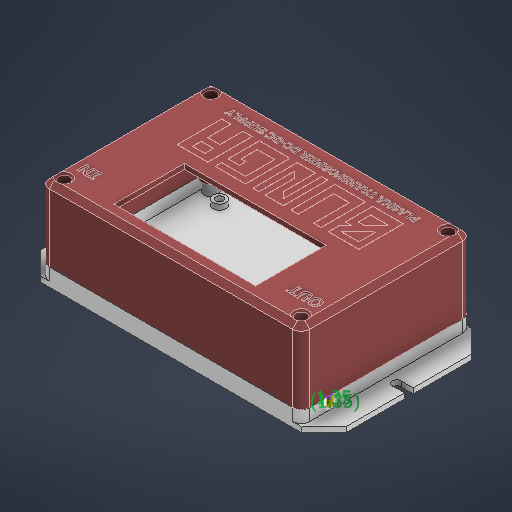
# Autodesk Inventor part: PowerSupplyCase-585W
Saved by Autodesk Inventor 2026.2 (Build 302298010, 298A)
## iProperties
Created: 2025-07-22
Part Number: PowerSupplyCase-585W
Material: Generic
Document SubType Name: Modeling
Designer: user
Density: 1 g/cm^3
Appearance: Default
Author: user
## iProperties of the stored document DrokSupplyCase_3DPrint.ipt
Created: 2025-07-22
Part Number: DrokSupplyCase_3DPrint
Material: Generic
Document SubType Name: Modeling
Designer: user
Density: 1 g/cm^3
Appearance: Default
Author: user
Autodesk Inventor part; units mm, degrees
(part 1 of 2)
sketch "Sketch1" plane through (0, 0, 0) normal (0, 1, 0) x (-1, 0, 0)
  line L0 (62, -35.75) -> (-62, -35.75) construction
  line L1 (-62, -35.75) -> (-62, 35.75) construction
  line L2 (-62, 35.75) -> (62, 35.75) construction
  line L3 (62, 35.75) -> (62, -35.75) construction
  line L4 (59, -32.775) -> (-59, -32.775) construction
  line L5 (-59, -32.775) -> (-59, 32.775) construction
  line L6 (-59, 32.775) -> (59, 32.775) construction
  line L7 (59, 32.775) -> (59, -32.775) construction
  circle A0 centre (59, -32.775) radius 2.1
  circle A1 centre (59, 32.775) radius 2.1
  circle A2 centre (-59, 32.775) radius 2.1
  circle A3 centre (-59, -32.775) radius 2.1
  circle A4 centre (59, -32.775) radius 3.75
  circle A5 centre (59, 32.775) radius 3.75
  circle A6 centre (-59, 32.775) radius 3.75
  circle A7 centre (-59, -32.775) radius 3.75
  line L8 (75, -43.75) -> (-75, -43.75)
  line L9 (-75, -43.75) -> (-75, 54.25)
  line L10 (-75, 54.25) -> (75, 54.25)
  line L11 (75, 54.25) -> (75, -43.75)
  line L12 (30.5, 5.75) -> (-48, 5.75)
  line L13 (-48, 5.75) -> (-48, 50.25)
  line L14 (-48, 50.25) -> (30.5, 50.25)
  line L15 (30.5, 50.25) -> (30.5, 5.75)
  line L16 (31.5, 21.85) -> (30.5, 21.85)
  line L17 (30.5, 21.85) -> (30.5, 34.15)
  line L18 (30.5, 34.15) -> (31.5, 34.15)
  line L19 (31.5, 34.15) -> (31.5, 21.85)
  line L20 (-48, 21.85) -> (-49, 21.85)
  line L21 (-49, 21.85) -> (-49, 34.15)
  line L22 (-49, 34.15) -> (-48, 34.15)
  line L23 (-48, 34.15) -> (-48, 21.85)
  line L24 (-72, -40.75) -> (72, -40.75)
  line L25 (72, -40.75) -> (72, 51.25)
  line L26 (72, 51.25) -> (-72, 51.25)
  line L27 (-72, 51.25) -> (-72, -40.75)
  line L28 (75, -43.75) -> (88, -30.75)
  line L29 (88, -30.75) -> (88, 41.25)
  line L30 (88, 41.25) -> (75, 54.25)
  circle A8 centre (81, 5.25) radius 2.5
  line L31 (81, 2.75) -> (88, 2.75)
  line L32 (81, 7.75) -> (88, 7.75)
  point P0 (0, 0)
  point P1 (0, -32.775)
  point P2 (0, -35.75)
  point P3 (-59, 0)
  point P4 (-62, 0)
  point P5 (30.5, 28)
  point P6 (-48, 28)
  point P7 (88, 5.25)
  point P8 (75, 5.25)
  dimension "d0" = 124
  dimension "d1" = 71.5
  dimension "d2" = 118
  dimension "d3" = 65.55
  dimension "d4" = 4.2
  dimension "d11" = 7.5
  dimension "d15" = 13
  dimension "d16" = 71.5
  dimension "d17" = 13
  dimension "d18" = 8
  dimension "d19" = 78.5
  dimension "d20" = 44.5
  dimension "d21" = 30
  dimension "d22" = 12.3
  dimension "d23" = 1
  dimension "d24" = 11
  dimension "d25" = 4
  dimension "d26" = 3
  dimension "d36" = 45
  dimension "d37" = 5
  dimension "d38" = 7
  dimension "d39" = 6
  constraints: 66 end point, 14 parallel, 10 midpoint, 9 centre point, 9 perpendicular, 8 coincident, 6 equal radius, 6 horizontal, 4 horizontal alignment, 2 equal length, 2 point on circle, 2 point on line, 2 tangent, 2 vertical alignment, 1 vertical, 3 other
  measures "d0" distance of L0.start L0.end
  measures "d1" distance of L2.end L0.start
  measures "d2" distance of L4.start L4.end
  measures "d3" distance of L6.end L4.start
  measures "d4" diameter of A0
  measures "d11" diameter of A4
  measures "d15" distance between parallel lines of L11 L3
  measures "d16" distance of L0.end L1.end
  measures "d17" distance between parallel lines of L9 L1
  measures "d18" distance between parallel lines of L8 L0
  measures "d19" distance of L12.start L12.end
  measures "d20" distance of L12.end L13.end
  measures "d21" distance between parallel lines of L12 L2
  measures "d22" distance of L18.end L16.start
  measures "d23" distance of L16.start L16.end
  measures "d24" distance between parallel lines of L5 L13
  measures "d25" distance between parallel lines of L10 L14
  measures "d26" distance between parallel lines of L8 L24
  measures "d36" angle of L28 L11
  measures "d37" diameter of A8
  measures "d38" distance of point (88, 5.25) A8.centre
  measures "d39" distance of point (75, 5.25) A8.centre
extrude "PCB Bosses" add sketch "Sketch1" along normal blind 6 contours A4 | A5 | A6 | A7
extrude "Floor" add sketch "Sketch1" along normal blind 3 contours A4 | A5 | A6 | A7 | L12 L13 L14 L15 | L15 L18 L19 L16 | L20 L21 L22 L13 | L27 L26 L25 L24
extrude "Fill in Holes" add sketch "Sketch1" along normal blind 1 contours A0 | A1 | A2 | A3
ref_plane "Work Plane1" through (-59, 49, -32.775) normal (0, 1, 0) x (1, 0, 0)
extrude "Wings" add sketch "Sketch1" along normal blind 3 contours L11 L30 L29 L32 A8 L31 L28
extrude "Bottom Wall" add sketch "Sketch1" along normal blind 3 contours L8 L9 L10 L11
mirror "Mirror1" about plane through (0, 0, 0) normal (1, 0, 0) of "Wings"
extrude "Bottom Wall 2" add sketch "Sketch1" along normal blind 10 contours L8 L9 L10 L11
fillet "Fillet1" radius 2 4 edges at (-72, 6.5, -40.75) (72, 6.5, -40.75) (-72, 6.5, 51.25) (72, 6.5, 51.25)
fillet "Fillet2" radius 5 4 edges at (-75, 6.5, 54.25) (75, 6.5, 54.25) (75, 6.5, -43.75) (-75, 6.5, -43.75)
sketch "Sketch2" plane through (0, 10, 0) normal (0, 1, 0) x (1, 0, 0)
  point P0 (0, 0)
sketch "Sketch3" plane through (0, 10, 0) normal (0, 1, 0) x (1, 0, 0)
  arc A0 (-70, 43.75) -> (-75, 38.75) centre (-70, 38.75) ccw projected
  line L0 (-75, 38.75) -> (-75, -49.25) projected
  arc A1 (-75, -49.25) -> (-70, -54.25) centre (-70, -49.25) ccw projected
  line L1 (-70, -54.25) -> (70, -54.25) projected
  arc A2 (70, -54.25) -> (75, -49.25) centre (70, -49.25) ccw projected
  line L2 (75, -49.25) -> (75, 38.75) projected
  arc A3 (75, 38.75) -> (70, 43.75) centre (70, 38.75) ccw projected
  line L3 (70, 43.75) -> (-70, 43.75) projected
  line L4 (72, 38.75) -> (72, -49.25) projected
  arc A4 (70, -51.25) -> (72, -49.25) centre (70, -49.25) ccw projected
  line L5 (70, -51.25) -> (-70, -51.25) projected
  arc A5 (-72, -49.25) -> (-70, -51.25) centre (-70, -49.25) ccw projected
  line L6 (-72, -49.25) -> (-72, 38.75) projected
  arc A6 (-70, 40.75) -> (-72, 38.75) centre (-70, 38.75) ccw projected
  line L7 (-70, 40.75) -> (70, 40.75) projected
  arc A7 (72, 38.75) -> (70, 40.75) centre (70, 38.75) ccw projected
  arc A8 (-70, 42.7) -> (-73.95, 38.75) centre (-70, 38.75) ccw
  line L8 (-70, 42.7) -> (70, 42.7)
  arc A9 (73.95, 38.75) -> (70, 42.7) centre (70, 38.75) ccw
  line L9 (73.95, 38.75) -> (73.95, -49.25)
  arc A10 (70, -53.2) -> (73.95, -49.25) centre (70, -49.25) ccw
  line L10 (70, -53.2) -> (-70, -53.2)
  arc A11 (-73.95, -49.25) -> (-70, -53.2) centre (-70, -49.25) ccw
  line L11 (-73.95, -49.25) -> (-73.95, 38.75)
  line L12 (70, 41.8) -> (-70, 41.8)
  arc A12 (-70, 41.8) -> (-73.05, 38.75) centre (-70, 38.75) ccw
  line L13 (-73.05, 38.75) -> (-73.05, -49.25)
  arc A13 (-73.05, -49.25) -> (-70, -52.3) centre (-70, -49.25) ccw
  line L14 (-70, -52.3) -> (70, -52.3)
  arc A14 (70, -52.3) -> (73.05, -49.25) centre (70, -49.25) ccw
  line L15 (73.05, -49.25) -> (73.05, 38.75)
  arc A15 (73.05, 38.75) -> (70, 41.8) centre (70, 38.75) ccw
  point P0 (0, 0)
  dimension "d48" = 1.05
  dimension "d49" = 1.05
  dimension "d50" = 0.9
  constraints: 16 end point, 16 point on circle, 8 centre point, 14 other
  measures "d48" radial gap between concentric circles of A0 A8
  measures "d49" distance between parallel lines of L7 L12
  measures "d50" distance between parallel lines of L12 L8
extrude "Lip 1" add sketch "Sketch3" along normal blind 1 contours L8 A9 L9 A10 L10 A11 L11 A8
sketch "Sketch4" plane through (-75, 3, -38.75) normal (-1, 0, 0) x (0, 0, 1)
  circle A0 centre (76.5, 3.35) radius 1.35
  line L0 (75.15, 2) -> (77.85, 2)
  line L1 (77.85, 2) -> (77.85, 8)
  line L2 (77.85, 8) -> (75.15, 8)
  line L3 (75.15, 8) -> (75.15, 2)
  line L4 (0, 8) -> (88, 8) projected
  line L5 (0, 7) -> (88, 7) projected
  line L6 (88, 7) -> (88, 0) projected
  line L7 (93, 0) -> (93, 7) projected
  point P0 (38.75, -3)
  point P1 (75.15, 3.35)
  point P2 (77.85, 3.35)
  dimension "d53" = 2.7
  dimension "d54" = 5
  dimension "d56" = 16.5
  constraints: 8 end point, 3 tangent, 2 parallel, 1 centre point, 1 collinear, 1 horizontal, 1 perpendicular
  measures "d53" diameter of A0
  measures "d54" distance between parallel lines of L5 L0
  measures "d56" distance from line of L7 A0.centre
sketch "Sketch5" plane through (0, 10, 0) normal (0, 1, 0) x (1, 0, 0)
  arc A0 (-70, 43.75) -> (-75, 38.75) centre (-70, 38.75) ccw projected
  line L0 (-75, 38.75) -> (-75, -49.25) projected
  arc A1 (-75, -49.25) -> (-70, -54.25) centre (-70, -49.25) ccw projected
  line L1 (-70, -54.25) -> (70, -54.25) projected
  arc A2 (70, -54.25) -> (75, -49.25) centre (70, -49.25) ccw projected
  line L2 (75, -49.25) -> (75, 38.75) projected
  arc A3 (75, 38.75) -> (70, 43.75) centre (70, 38.75) ccw projected
  line L3 (70, 43.75) -> (-70, 43.75) projected
  arc A4 (73.95, 38.75) -> (70, 42.7) centre (70, 38.75) ccw projected
  line L4 (73.95, 38.75) -> (73.95, -49.25) projected
  arc A5 (70, -53.2) -> (73.95, -49.25) centre (70, -49.25) ccw projected
  line L5 (70, -53.2) -> (-70, -53.2) projected
  arc A6 (-73.95, -49.25) -> (-70, -53.2) centre (-70, -49.25) ccw projected
  line L6 (-73.95, -49.25) -> (-73.95, 38.75) projected
  arc A7 (-70, 42.7) -> (-73.95, 38.75) centre (-70, 38.75) ccw projected
  line L7 (-70, 42.7) -> (70, 42.7) projected
  line L8 (70, 41.8) -> (-70, 41.8) projected
  arc A8 (-70, 41.8) -> (-73.05, 38.75) centre (-70, 38.75) ccw projected
  line L9 (-73.05, 38.75) -> (-73.05, -49.25) projected
  arc A9 (-73.05, -49.25) -> (-70, -52.3) centre (-70, -49.25) ccw projected
  line L10 (-70, -52.3) -> (70, -52.3) projected
  arc A10 (70, -52.3) -> (73.05, -49.25) centre (70, -49.25) ccw projected
  line L11 (73.05, -49.25) -> (73.05, 38.75) projected
  arc A11 (73.05, 38.75) -> (70, 41.8) centre (70, 38.75) ccw projected
  line L12 (72, 38.75) -> (72, -49.25) projected
  arc A12 (70, -51.25) -> (72, -49.25) centre (70, -49.25) ccw projected
  line L13 (70, -51.25) -> (-70, -51.25) projected
  arc A13 (-72, -49.25) -> (-70, -51.25) centre (-70, -49.25) ccw projected
  line L14 (-72, -49.25) -> (-72, 38.75) projected
  arc A14 (-70, 40.75) -> (-72, 38.75) centre (-70, 38.75) ccw projected
  line L15 (-70, 40.75) -> (70, 40.75) projected
  arc A15 (72, 38.75) -> (70, 40.75) centre (70, 38.75) ccw projected
  line L16 (-74.1, 38.75) -> (-74.1, -49.25)
  arc A16 (-74.1, -49.25) -> (-70, -53.35) centre (-70, -49.25) ccw
  line L17 (-70, -53.35) -> (70, -53.35)
  arc A17 (70, -53.35) -> (74.1, -49.25) centre (70, -49.25) ccw
  line L18 (74.1, -49.25) -> (74.1, 38.75)
  arc A18 (74.1, 38.75) -> (70, 42.85) centre (70, 38.75) ccw
  line L19 (70, 42.85) -> (-70, 42.85)
  arc A19 (-70, 42.85) -> (-74.1, 38.75) centre (-70, 38.75) ccw
  arc A20 (-70, 41.65) -> (-72.9, 38.75) centre (-70, 38.75) ccw
  line L20 (-70, 41.65) -> (70, 41.65)
  arc A21 (72.9, 38.75) -> (70, 41.65) centre (70, 38.75) ccw
  line L21 (72.9, 38.75) -> (72.9, -49.25)
  arc A22 (70, -52.15) -> (72.9, -49.25) centre (70, -49.25) ccw
  line L22 (70, -52.15) -> (-70, -52.15)
  arc A23 (-72.9, -49.25) -> (-70, -52.15) centre (-70, -49.25) ccw
  line L23 (-72.9, -49.25) -> (-72.9, 38.75)
  point P0 (0, 0)
  dimension "d59" = 0.15
  dimension "d60" = 0.15
  constraints: 16 end point, 16 point on circle, 8 centre point, 14 other
  measures "d59" radial gap between concentric circles of A7 A19
  measures "d60" radial gap between concentric circles of A8 A20
extrude "Extrusion10" add sketch "Sketch5" along normal blind 1.1 separate body contours L3 A3 L2 A2 L1 A1 L0 A0 | L20 A21 L21 A22 L22 A23 L23 A20
sketch "Sketch6" plane through (0, 11.1, 0) normal (0, 1, 0) x (1, 0, 0)
  line L0 (-75, 38.75) -> (-75, -49.25) projected
  arc A0 (-75, -49.25) -> (-70, -54.25) centre (-70, -49.25) ccw projected
  line L1 (-70, -54.25) -> (70, -54.25) projected
  arc A1 (70, -54.25) -> (75, -49.25) centre (70, -49.25) ccw projected
  line L2 (75, -49.25) -> (75, 38.75) projected
  arc A2 (75, 38.75) -> (70, 43.75) centre (70, 38.75) ccw projected
  line L3 (70, 43.75) -> (-70, 43.75) projected
  arc A3 (-70, 43.75) -> (-75, 38.75) centre (-70, 38.75) ccw projected
  arc A4 (-70, 42.85) -> (-74.1, 38.75) centre (-70, 38.75) ccw projected
  line L4 (-70, 42.85) -> (70, 42.85) projected
  arc A5 (74.1, 38.75) -> (70, 42.85) centre (70, 38.75) ccw projected
  line L5 (74.1, 38.75) -> (74.1, -49.25) projected
  arc A6 (70, -53.35) -> (74.1, -49.25) centre (70, -49.25) ccw projected
  line L6 (70, -53.35) -> (-70, -53.35) projected
  arc A7 (-74.1, -49.25) -> (-70, -53.35) centre (-70, -49.25) ccw projected
  line L7 (-74.1, -49.25) -> (-74.1, 38.75) projected
  line L8 (70, 41.65) -> (-70, 41.65) projected
  arc A8 (-70, 41.65) -> (-72.9, 38.75) centre (-70, 38.75) ccw projected
  line L9 (-72.9, 38.75) -> (-72.9, -49.25) projected
  arc A9 (-72.9, -49.25) -> (-70, -52.15) centre (-70, -49.25) ccw projected
  line L10 (-70, -52.15) -> (70, -52.15) projected
  arc A10 (70, -52.15) -> (72.9, -49.25) centre (70, -49.25) ccw projected
  line L11 (72.9, -49.25) -> (72.9, 38.75) projected
  arc A11 (72.9, 38.75) -> (70, 41.65) centre (70, 38.75) ccw projected
  line L12 (-70, 40.75) -> (70, 40.75) projected
  arc A12 (72, 38.75) -> (70, 40.75) centre (70, 38.75) ccw projected
  line L13 (72, 38.75) -> (72, -49.25) projected
  arc A13 (70, -51.25) -> (72, -49.25) centre (70, -49.25) ccw projected
  line L14 (70, -51.25) -> (-70, -51.25) projected
  arc A14 (-72, -49.25) -> (-70, -51.25) centre (-70, -49.25) ccw projected
  line L15 (-72, -49.25) -> (-72, 38.75) projected
  arc A15 (-70, 40.75) -> (-72, 38.75) centre (-70, 38.75) ccw projected
  point P0 (0, 0)
extrude "Extrusion11" add sketch "Sketch6" along normal up to surface (37.9 mm away) contours A3 L3 A2 L2 A1 L1 A0 L0 | L4 A5 L5 A6 L6 A7 L7 A4 | A11 L11 A10 L10 A9 L9 A8 L8 bodies 2
sketch "Sketch7" plane through (-70, 49, 54.25) normal (0, 1, 0) x (1, 0, 0)
  line L0 (39.5, 48.5) -> (118, 48.5) projected
  line L1 (39.5, 4) -> (39.5, 48.5) projected
  line L2 (118, 4) -> (39.5, 4) projected
  line L3 (118, 48.5) -> (118, 4) projected
  line L4 (119, 20.1) -> (118, 20.1) projected
  line L5 (119, 32.4) -> (119, 20.1) projected
  line L6 (118, 32.4) -> (119, 32.4) projected
  line L7 (39.5, 20.1) -> (38.5, 20.1) projected
  line L8 (38.5, 20.1) -> (38.5, 32.4) projected
  line L9 (38.5, 32.4) -> (39.5, 32.4) projected
  arc A0 (-2, 5) -> (0, 3) centre (0, 5) ccw projected
  line L10 (-2, 93) -> (-2, 5) projected
  arc A1 (0, 95) -> (-2, 93) centre (0, 93) ccw projected
  line L11 (140, 95) -> (0, 95) projected
  arc A2 (142, 93) -> (140, 95) centre (140, 93) ccw projected
  line L12 (142, 5) -> (142, 93) projected
  arc A3 (140, 3) -> (142, 5) centre (140, 5) ccw projected
  line L13 (0, 3) -> (140, 3) projected
  line L14 (-5, 5) -> (-5, 93) projected
  arc A4 (-5, 5) -> (0, 0) centre (0, 5) ccw projected
  line L15 (140, 0) -> (0, 0) projected
  arc A5 (140, 0) -> (145, 5) centre (140, 5) ccw projected
  line L16 (145, 93) -> (145, 5) projected
  arc A6 (145, 93) -> (140, 98) centre (140, 93) ccw projected
  line L17 (0, 98) -> (140, 98) projected
  arc A7 (0, 98) -> (-5, 93) centre (0, 93) ccw projected
  point P0 (70, 54.25)
extrude "Extrusion12" add sketch "Sketch7" along normal blind 3 contours L10 A1 L11 A2 L12 A3 L13 A0 | L14 A7 L17 A6 L16 A5 L15 A4 bodies 2
sketch "Sketch8" plane through (0, 3, 0) normal (0, 1, 0) x (1, 0, 0)
  circle A0 centre (-68.25, 37) radius 2.1
  circle A1 centre (-68.25, 37) radius 3.75
  circle A2 centre (59, -32.775) radius 3.75 projected
  circle A3 centre (59, 32.775) radius 3.75 projected
  circle A4 centre (-59, -32.775) radius 3.75 projected
  circle A5 centre (-59, 32.775) radius 3.75 projected
  arc A6 (70, -51.25) -> (72, -49.25) centre (70, -49.25) ccw projected
  line L0 (72, -49.25) -> (72, 38.75) projected
  arc A7 (72, 38.75) -> (70, 40.75) centre (70, 38.75) ccw projected
  line L1 (70, 40.75) -> (-70, 40.75) projected
  arc A8 (-70, 40.75) -> (-72, 38.75) centre (-70, 38.75) ccw projected
  line L2 (-72, 38.75) -> (-72, -49.25) projected
  arc A9 (-72, -49.25) -> (-70, -51.25) centre (-70, -49.25) ccw projected
  line L3 (-70, -51.25) -> (70, -51.25) projected
  line L4 (-70, 40.75) -> (70, 40.75) projected
  line L5 (-72, -49.25) -> (-72, 38.75) projected
  circle A10 centre (-68.25, -47.5) radius 2.1
  circle A11 centre (-68.25, -47.5) radius 3.75
  circle A12 centre (68.25, -47.5) radius 2.1
  circle A13 centre (68.25, -47.5) radius 3.75
  circle A14 centre (68.25, 37) radius 2.1
  circle A15 centre (68.25, 37) radius 3.75
  line L6 (70, -51.25) -> (-70, -51.25) projected
  line L7 (72, 38.75) -> (72, -49.25) projected
  point P0 (0, 0)
  dimension "d69" = 4.2
  dimension "d70" = 7.5
  constraints: 8 centre point, 8 tangent, 6 equal radius, 4 coincident
  measures "d69" diameter of A0
  measures "d70" diameter of A1
extrude "Extrusion13" add sketch "Sketch8" along normal up to surface (7 mm away) contours A1 | A15 | A11 | A13 bodies 1
sketch "Sketch9" plane through (-68.25, 3, -37) normal (0, 1, 0) x (1, 0, 0)
  circle A0 centre (0, 0) radius 2.1 projected
  circle A1 centre (136.5, 0) radius 2.1 projected
  circle A2 centre (136.5, -84.5) radius 2.1 projected
  circle A3 centre (0, -84.5) radius 2.1 projected
  point P0 (68.25, -37)
extrude "Extrusion14" cut sketch "Sketch9" against normal blind 2 bodies 1
extrude "Extrusion15" cut sketch "Sketch4" against normal up to surface (150 mm away) contours A0 | A0 L3 L5 L1 | L5 L3 L2 L1 bodies 1
sketch "Sketch10" plane through (-70, 52, 54.25) normal (0, 1, 0) x (1, 0, 0)
  arc A0 (1.75, 95) -> (-2, 91.25) centre (1.75, 91.25) ccw construction
  arc A1 (-2, 91.25) -> (1.75, 95) centre (1.75, 91.25) ccw construction
  circle A2 centre (1.75, 91.25) radius 2.1 construction
  circle A3 centre (138.25, 91.25) radius 2.1 construction
  arc A4 (138.25, 95) -> (142, 91.25) centre (138.25, 91.25) ccw construction
  arc A5 (142, 91.25) -> (138.25, 95) centre (138.25, 91.25) ccw construction
  circle A6 centre (138.25, 6.75) radius 2.1 construction
  arc A7 (142, 6.75) -> (138.25, 3) centre (138.25, 6.75) ccw construction
  arc A8 (138.25, 3) -> (142, 6.75) centre (138.25, 6.75) ccw construction
  arc A9 (1.75, 3) -> (-2, 6.75) centre (1.75, 6.75) ccw construction
  arc A10 (-2, 6.75) -> (1.75, 3) centre (1.75, 6.75) ccw construction
  circle A11 centre (1.75, 6.75) radius 2.1 construction
  circle A12 centre (1.75, 91.25) radius 1.7
  circle A13 centre (1.75, 91.25) radius 3.25
  circle A14 centre (1.75, 91.25) radius 5.25
  point P0 (70, 54.25)
  dimension "d81" = 3.4
  dimension "d82" = 6.5
  dimension "d83" = 2
  constraints: 3 centre point, 2 coincident
  measures "d81" diameter of A12
  measures "d82" diameter of A13
  measures "d83" radial gap between concentric circles of A13 A14
sketch "Sketch11" plane through (-70, 49, 54.25) normal (0, -1, 0) x (1, 0, 0)
  circle A0 centre (1.75, -91.25) radius 5.25 projected
  line L0 (-5, -93) -> (-5, -5) projected
  line L1 (-5, -93) -> (-5, -5) projected
  arc A1 (-5, -93) -> (0, -98) centre (0, -93) ccw projected
  line L2 (140, -98) -> (0, -98) projected
  line L3 (140, -98) -> (0, -98) projected
  line L4 (140, -95.9) -> (0, -95.9) projected
  arc A2 (140, -95.9) -> (142.9, -93) centre (140, -93) ccw projected
  line L5 (142.9, -5) -> (142.9, -93) projected
  arc A3 (142.9, -5) -> (140, -2.1) centre (140, -5) ccw projected
  line L6 (0, -2.1) -> (140, -2.1) projected
  arc A4 (0, -2.1) -> (-2.9, -5) centre (0, -5) ccw projected
  line L7 (-2.9, -93) -> (-2.9, -5) projected
  arc A5 (-2.9, -93) -> (0, -95.9) centre (0, -93) ccw projected
  line L8 (0, -95) -> (140, -95) projected
  arc A6 (-2, -93) -> (0, -95) centre (0, -93) ccw projected
  line L9 (-2, -5) -> (-2, -93) projected
  arc A7 (0, -3) -> (-2, -5) centre (0, -5) ccw projected
  line L10 (140, -3) -> (0, -3) projected
  arc A8 (142, -5) -> (140, -3) centre (140, -5) ccw projected
  line L11 (142, -93) -> (142, -5) projected
  arc A9 (140, -95) -> (142, -93) centre (140, -93) ccw projected
  arc A10 (-5, -93) -> (0, -98) centre (0, -93) ccw projected
  point P0 (70, -54.25)
  point P1 (5.4242, -95)
  point P2 (-2, -87.5758)
extrude "TopMount1" add sketch "Sketch11" along normal up to surface (39 mm away) contours A0 L8 A6 L9 bodies 2
extrude "TopMount2" cut sketch "Sketch10" against normal up to surface (42 mm away) contours A12 bodies 2
ref_plane "Work Plane2" through (0, 12, 0) normal (0, -1, 0) x (1, 0, 0)
extrude "TopMount3" cut sketch "Sketch10" against normal up to surface (40 mm away) contours A13 bodies 2
ref_plane "Work Plane3" through (0, 10, 49.25) normal (1, 0, 0) x (0, 0, -1)
ref_plane "Work Plane4" through (-70, 10, 5.25) normal (0, 0, 1) x (1, 0, 0)
mirror "Mirror2" about plane through (0, 10, 49.25) normal (1, 0, 0) of "TopMount3", "TopMount2", "TopMount1" bodies 2
mirror "Mirror3" about plane through (-70, 10, 5.25) normal (0, 0, 1) of "TopMount3", "TopMount2", "TopMount1", "Mirror2" bodies 2
sketch "Sketch12" plane through (-70, 52, 54.25) normal (0, 1, 0) x (1, 0, 0)
  line L0 (78.75, 56) -> (61.25, 56) construction
  line L1 (61.25, 56) -> (61.25, 81.5) construction
  line L2 (61.25, 81.5) -> (78.75, 81.5) construction
  line L3 (78.75, 81.5) -> (78.75, 56) construction
  line L4 (57, 56) -> (39.5, 56) construction
  line L5 (57, 81.5) -> (57, 56) construction
  line L6 (39.5, 81.5) -> (57, 81.5) construction
  line L7 (39.5, 56) -> (39.5, 81.5) construction
  line L8 (35.25, 56) -> (17.75, 56) construction
  line L9 (35.25, 81.5) -> (35.25, 56) construction
  line L10 (17.75, 81.5) -> (35.25, 81.5) construction
  line L11 (17.75, 56) -> (17.75, 81.5) construction
  line L12 (100.5, 56) -> (83, 56) construction
  line L13 (100.5, 81.5) -> (100.5, 56) construction
  line L14 (83, 81.5) -> (100.5, 81.5) construction
  line L15 (83, 56) -> (83, 81.5) construction
  line L16 (78.75, 56) -> (61.25, 56) construction
  line L17 (78.75, 81.5) -> (78.75, 56) construction
  line L18 (61.25, 81.5) -> (78.75, 81.5) construction
  line L19 (61.25, 56) -> (61.25, 81.5) construction
  line L20 (57, 56) -> (39.5, 56) construction
  line L21 (57, 81.5) -> (57, 56) construction
  line L22 (39.5, 81.5) -> (57, 81.5) construction
  line L23 (39.5, 56) -> (39.5, 81.5) construction
  line L24 (122.25, 56) -> (104.75, 56) construction
  line L25 (122.25, 81.5) -> (122.25, 56) construction
  line L26 (104.75, 81.5) -> (122.25, 81.5) construction
  line L27 (104.75, 56) -> (104.75, 81.5) construction
  line L28 (100.5, 56) -> (83, 56) construction
  line L29 (100.5, 81.5) -> (100.5, 56) construction
  line L30 (83, 81.5) -> (100.5, 81.5) construction
  line L31 (83, 56) -> (83, 81.5) construction
  line L32 (78.75, 56) -> (61.25, 56) construction
  line L33 (78.75, 81.5) -> (78.75, 56) construction
  line L34 (61.25, 81.5) -> (78.75, 81.5) construction
  line L35 (61.25, 56) -> (61.25, 81.5) construction
  line L36 (78.75, 81.5) -> (78.75, 56)
  line L37 (68.25, 56) -> (68.25, 73)
  line L38 (68.25, 73) -> (64.75, 76.5)
  line L39 (64.75, 76.5) -> (64.75, 56)
  line L40 (61.25, 56) -> (61.25, 81.5)
  line L41 (61.25, 81.5) -> (71.75, 81.5)
  line L42 (71.75, 81.5) -> (71.75, 63.25)
  line L43 (71.75, 63.25) -> (75.25, 59.75)
  line L44 (75.25, 59.75) -> (75.25, 81.5)
  line L45 (75.25, 81.5) -> (78.75, 81.5)
  line L46 (39.5, 56) -> (57, 56)
  line L47 (57, 56) -> (57, 81.5)
  line L48 (57, 81.5) -> (39.5, 81.5)
  line L49 (39.5, 81.5) -> (39.5, 63.5)
  line L50 (39.5, 63.5) -> (46, 63.5)
  line L51 (46, 63.5) -> (46, 67.25)
  line L52 (46, 67.25) -> (43.25, 67.25)
  line L53 (43.25, 67.25) -> (43.25, 76.5)
  line L54 (43.25, 76.5) -> (53.25, 76.5)
  line L55 (53.25, 76.5) -> (53.25, 59.75)
  line L56 (53.25, 59.75) -> (39.5, 59.75)
  line L57 (39.5, 59.75) -> (39.5, 56)
  line L58 (35.25, 81.5) -> (30, 81.5)
  line L59 (30, 81.5) -> (30, 68.25)
  line L60 (30, 68.25) -> (23, 68.25)
  line L61 (23, 68.25) -> (23, 81.5)
  line L62 (23, 81.5) -> (17.75, 81.5)
  line L63 (17.75, 81.5) -> (17.75, 56)
  line L64 (17.75, 56) -> (35.25, 56)
  line L65 (35.25, 56) -> (35.25, 81.5)
  line L66 (30, 59.5) -> (30, 64.5)
  line L67 (30, 64.5) -> (23, 64.5)
  line L68 (23, 64.5) -> (23, 59.5)
  line L69 (23, 59.5) -> (30, 59.5)
  line L70 (100.5, 56) -> (96.25, 56)
  line L71 (96.25, 56) -> (96.25, 76.5)
  line L72 (96.25, 76.5) -> (87.25, 76.5)
  line L73 (87.25, 76.5) -> (87.25, 56)
  line L74 (83, 56) -> (83, 81.5)
  line L75 (83, 81.5) -> (100.5, 81.5)
  line L76 (100.5, 81.5) -> (100.5, 56)
  line L77 (122.25, 56) -> (122.25, 81.5)
  line L78 (122.25, 81.5) -> (104.75, 81.5)
  line L79 (104.75, 56) -> (122.25, 56)
  line L80 (118.5, 59.75) -> (118.5, 69.031)
  line L81 (118.5, 64.3905) -> (111.5898, 64.3905) construction
  line L82 (107.3101, 68.75) -> (104.75, 68.75) construction
  line L83 (118.5, 69.031) -> (117.1257, 69.031)
  line L84 (117.1257, 69.031) -> (108.5, 60.4053)
  line L85 (117.1257, 69.031) -> (129.3242, 69.031) construction
  line L86 (108.5, 60.4053) -> (108.5, 59.75)
  line L87 (108.5, 59.75) -> (118.5, 59.75)
  line L88 (107.3101, 68.75) -> (104.75, 68.75) construction
  line L89 (112.25, 69.4886) -> (108.5, 69.4886)
  line L90 (108.5, 69.4886) -> (108.5, 76.5)
  line L91 (108.5, 76.5) -> (118.5, 76.5)
  line L92 (118.5, 76.5) -> (118.5, 75.7386)
  line L93 (118.5, 75.7386) -> (112.25, 69.4886)
  line L94 (118.5, 75.7386) -> (125.6277, 75.7386) construction
  line L95 (104.75, 56) -> (104.75, 61.9886)
  line L96 (104.75, 61.9886) -> (108.5, 65.7386)
  line L97 (108.5, 65.7386) -> (104.75, 65.7386)
  line L98 (104.75, 81.5) -> (104.75, 65.7386)
  line L99 (108.5, 65.7386) -> (112.25, 69.4886) construction
  line L100 (5, 93) -> (135, 93) projected
  line L101 (70, 93) -> (70, 48.5) construction
  line L102 (39.5, 48.5) -> (118, 48.5) construction
  line L103 (61.25, 56) -> (64.75, 56)
  line L104 (68.25, 56) -> (78.75, 56)
  line L105 (83, 56) -> (87.25, 56)
  point P0 (70, 54.25)
  point P1 (70, 68.75)
  point P2 (60, 68.75)
  point P3 (70, 56)
  point P4 (61.25, 68.75)
  point P5 (48.25, 56)
  point P6 (48.25, 68.75)
  point P7 (39.5, 68.75)
  point P8 (26.5, 56)
  point P9 (26.5, 68.75)
  point P10 (17.75, 68.75)
  point P11 (91.75, 56)
  point P12 (91.75, 68.75)
  point P13 (83, 68.75)
  point P14 (70, 56)
  point P15 (70, 68.75)
  point P16 (61.25, 68.75)
  point P17 (48.25, 56)
  point P18 (48.25, 68.75)
  point P19 (39.5, 68.75)
  point P20 (113.5, 56)
  point P21 (113.5, 68.75)
  point P22 (91.75, 56)
  point P23 (91.75, 68.75)
  point P24 (83, 68.75)
  point P25 (70, 56)
  point P26 (70, 68.75)
  point P27 (61.25, 68.75)
  point P28 (107.3101, 68.75)
  point P29 (102.125, 63.5649)
  point P30 (70, 68.75)
  point P31 (70, 70.75)
  point P32 (5, 91.25)
  point P33 (135, 91.25)
  point P34 (70, 70.75)
  constraints: 208 end point, 27 perpendicular, 18 point on line, 17 collinear, 9 horizontal, 6 midpoint, 6 vertical, 4 parallel, 3 horizontal alignment, 2 coincident, 2 vertical alignment, 1 equal length, 6 other
extrude "Extrusion19" cut sketch "Sketch12" against normal blind 0.1 bodies 2
sketch "Sketch13" plane through (-70, 52, 54.25) normal (0, 1, 0) x (1, 0, 0)
  line L0 (139.3009, 14) -> (124.6991, 14) construction
  line L1 (124.6991, 14) -> (124.6991, 17.3208) construction
  line L2 (124.6991, 17.3208) -> (139.3009, 17.3208) construction
  line L3 (139.3009, 17.3208) -> (139.3009, 14) construction
  line L4 (141.5993, 14) -> (126.9975, 14) construction
  line L5 (126.9975, 14) -> (126.9975, 17.3208) construction
  line L6 (126.9975, 17.3208) -> (141.5993, 17.3208) construction
  line L7 (141.5993, 17.3208) -> (141.5993, 14) construction
  line L8 (11.2814, 14) -> (-3.3204, 14) construction
  line L9 (-3.3204, 14) -> (-3.3204, 17.3208) construction
  line L10 (-3.3204, 17.3208) -> (11.2814, 17.3208) construction
  line L11 (11.2814, 17.3208) -> (11.2814, 14) construction
  line L12 (140, 91.25) -> (140, 6.75) projected
  line L13 (134, 5) -> (117.75, 5) projected
  line L14 (136.0195, 85.116) -> (3.9805, 85.116) construction
  line L15 (3.9805, 85.116) -> (3.9805, 87.6939) construction
  line L16 (3.9805, 87.6939) -> (136.0195, 87.6939) construction
  line L17 (136.0195, 87.6939) -> (136.0195, 85.116) construction
  line L18 (6, 93) -> (134, 93) projected
  spline S0 degree 2 poles (133.2239, 17.1235) (133.2239, 18.5808) (134.7784, 20.247) (136.1288, 20.247) knots 0 0 0 1 2 2 2
  spline S1 degree 2 poles (136.1288, 20.247) (137.4841, 20.247) (139.0289, 18.5614) (139.0289, 17.1235) knots 0 0 0 1 2 2 2
  spline S2 degree 2 poles (139.0289, 17.1235) (139.0289, 15.6808) (137.4841, 14) (136.1288, 14) knots 0 0 0 1 2 2 2
  spline S3 degree 2 poles (136.1288, 14) (134.7784, 14) (133.2239, 15.671) (133.2239, 17.1235) knots 0 0 0 1 2 2 2
  spline S4 degree 2 poles (134.7784, 17.1235) (134.7784, 16.5843) (134.997, 15.8314) (135.1865, 15.5933) knots 0 0 0 1 2 2 2
  spline S5 degree 2 poles (135.1865, 15.5933) (135.3759, 15.3456) (135.8617, 15.1318) (136.124, 15.1318) knots 0 0 0 1 2 2 2
  spline S6 degree 2 poles (136.124, 15.1318) (136.4009, 15.1318) (136.8526, 15.331) (137.0615, 15.5836) knots 0 0 0 1 2 2 2
  spline S7 degree 2 poles (137.0615, 15.5836) (137.2461, 15.8168) (137.4744, 16.5892) (137.4744, 17.1235) knots 0 0 0 1 2 2 2
  spline S8 degree 2 poles (137.4744, 17.1235) (137.4744, 17.6773) (137.2558, 18.4059) (137.0664, 18.6537) knots 0 0 0 1 2 2 2
  spline S9 degree 2 poles (137.0664, 18.6537) (136.8769, 18.9014) (136.3863, 19.1152) (136.124, 19.1152) knots 0 0 0 1 2 2 2
  spline S10 degree 2 poles (136.124, 19.1152) (135.8568, 19.1152) (135.3613, 18.8868) (135.1816, 18.644) knots 0 0 0 1 2 2 2
  spline S11 degree 2 poles (135.1816, 18.644) (134.9873, 18.3816) (134.7784, 17.687) (134.7784, 17.1235) knots 0 0 0 1 2 2 2
  spline S12 degree 2 poles (129.9061, 20.247) (131.1157, 20.247) (132.4176, 19.0812) (132.4176, 17.9542) knots 0 0 0 1 2 2 2
  line L19 (132.4176, 17.9542) -> (132.4176, 14.1263)
  line L20 (132.4176, 14.1263) -> (130.9117, 14.1263)
  line L21 (130.9117, 14.1263) -> (130.9117, 17.8667)
  spline S13 degree 2 poles (130.9117, 17.8667) (130.9117, 18.4934) (130.4405, 19.1054) (129.9061, 19.1054) knots 0 0 0 1 2 2 2
  spline S14 degree 2 poles (129.9061, 19.1054) (129.3864, 19.1054) (128.9006, 18.5177) (128.9006, 17.8667) knots 0 0 0 1 2 2 2
  line L22 (128.9006, 17.8667) -> (128.9006, 14.1263)
  line L23 (128.9006, 14.1263) -> (127.3947, 14.1263)
  line L24 (127.3947, 14.1263) -> (127.3947, 17.9493)
  spline S15 degree 2 poles (127.3947, 17.9493) (127.3947, 19.0569) (128.6626, 20.247) (129.9061, 20.247) knots 0 0 0 1 2 2 2
  line L25 (125.0873, 20.1207) -> (125.0873, 15.2679)
  line L26 (125.0873, 15.2679) -> (126.8604, 15.2679)
  line L27 (126.8604, 15.2679) -> (126.8604, 14.1263)
  line L28 (126.8604, 14.1263) -> (121.8084, 14.1263)
  line L29 (121.8084, 14.1263) -> (121.8084, 15.2679)
  line L30 (121.8084, 15.2679) -> (123.5814, 15.2679)
  line L31 (123.5814, 15.2679) -> (123.5814, 20.1207)
  line L32 (123.5814, 20.1207) -> (125.0873, 20.1207)
  line L33 (7.677, 19.9944) -> (10.9025, 19.9944)
  line L34 (10.9025, 19.9944) -> (10.9025, 18.95)
  line L35 (10.9025, 18.95) -> (10.0427, 18.95)
  line L36 (10.0427, 18.95) -> (10.0427, 15.0444)
  line L37 (10.0427, 15.0444) -> (10.9025, 15.0444)
  line L38 (10.9025, 15.0444) -> (10.9025, 14)
  line L39 (10.9025, 14) -> (7.677, 14)
  line L40 (7.677, 14) -> (7.677, 15.0444)
  line L41 (7.677, 15.0444) -> (8.5368, 15.0444)
  line L42 (8.5368, 15.0444) -> (8.5368, 18.95)
  line L43 (8.5368, 18.95) -> (7.677, 18.95)
  line L44 (7.677, 18.95) -> (7.677, 19.9944)
  line L45 (1.5417, 19.9944) -> (2.9893, 19.9944)
  line L46 (2.9893, 19.9944) -> (5.3016, 15.8168)
  line L47 (5.3016, 15.8168) -> (5.3016, 19.9944)
  line L48 (5.3016, 19.9944) -> (6.6763, 19.9944)
  line L49 (6.6763, 19.9944) -> (6.6763, 14)
  line L50 (6.6763, 14) -> (4.8304, 14)
  line L51 (4.8304, 14) -> (2.9165, 17.4344)
  line L52 (2.9165, 17.4344) -> (2.9165, 14)
  line L53 (2.9165, 14) -> (1.5417, 14)
  line L54 (1.5417, 14) -> (1.5417, 19.9944)
  spline S16 degree 2 poles (121.2823, 86.4571) (121.2823, 86.735) (121.4601, 87.2392) (121.6249, 87.4072) knots 0 0 0 1 2 2 2
  spline S17 degree 2 poles (121.6249, 87.4072) (121.7251, 87.5139) (121.9707, 87.6884) (122.1161, 87.7498) knots 0 0 0 1 2 2 2
  spline S18 degree 2 poles (122.1161, 87.7498) (122.2647, 87.8112) (122.6105, 87.8823) (122.8238, 87.8823) knots 0 0 0 1 2 2 2
  line L55 (122.8238, 87.8823) -> (123.3473, 87.8823)
  line L56 (123.3473, 87.8823) -> (123.3473, 89.1878)
  line L57 (123.3473, 89.1878) -> (124.3491, 89.1878)
  line L58 (124.3491, 89.1878) -> (124.3491, 85.2)
  line L59 (124.3491, 85.2) -> (122.8012, 85.2)
  spline S19 degree 2 poles (122.8012, 85.2) (122.4586, 85.2) (121.9577, 85.3261) (121.7541, 85.4618) knots 0 0 0 1 2 2 2
  spline S20 degree 2 poles (121.7541, 85.4618) (121.5279, 85.6137) (121.2823, 86.1113) (121.2823, 86.4571) knots 0 0 0 1 2 2 2
  spline S21 degree 2 poles (122.31, 86.483) (122.31, 86.3117) (122.4716, 86.0693) (122.5814, 86.0241) knots 0 0 0 1 2 2 2
  spline S22 degree 2 poles (122.5814, 86.0241) (122.7236, 85.9627) (122.9822, 85.9433) (123.2051, 85.9433) knots 0 0 0 1 2 2 2
  line L60 (123.2051, 85.9433) -> (123.3473, 85.9433)
  line L61 (123.3473, 85.9433) -> (123.3473, 87.139)
  line L62 (123.3473, 87.139) -> (123.2762, 87.139)
  spline S23 degree 2 poles (123.2762, 87.139) (123.1373, 87.139) (122.8852, 87.1325) (122.7915, 87.1164) knots 0 0 0 1 2 2 2
  spline S24 degree 2 poles (122.7915, 87.1164) (122.7107, 87.1034) (122.533, 87.0259) (122.4845, 86.9774) knots 0 0 0 1 2 2 2
  spline S25 degree 2 poles (122.4845, 86.9774) (122.3811, 86.8805) (122.31, 86.6639) (122.31, 86.483) knots 0 0 0 1 2 2 2
  line L63 (118.0863, 89.1878) -> (120.7459, 89.1878)
  line L64 (120.7459, 89.1878) -> (120.7459, 85.2)
  line L65 (120.7459, 85.2) -> (119.7441, 85.2)
  line L66 (119.7441, 85.2) -> (119.7441, 88.4284)
  line L67 (119.7441, 88.4284) -> (118.0863, 88.4284)
  line L68 (118.0863, 88.4284) -> (118.0863, 89.1878)
  line L69 (118.0378, 89.1878) -> (116.6902, 85.2)
  line L70 (116.6902, 85.2) -> (115.5979, 85.2)
  line L71 (115.5979, 85.2) -> (114.2504, 89.1878)
  line L72 (114.2504, 89.1878) -> (115.2812, 89.1878)
  line L73 (115.2812, 89.1878) -> (115.5301, 88.3735)
  line L74 (115.5301, 88.3735) -> (116.7839, 88.3735)
  line L75 (116.7839, 88.3735) -> (117.036, 89.1878)
  line L76 (117.036, 89.1878) -> (118.0378, 89.1878)
  line L77 (115.7498, 87.6496) -> (116.157, 86.3311)
  line L78 (116.157, 86.3311) -> (116.5674, 87.6496)
  line L79 (116.5674, 87.6496) -> (115.7498, 87.6496)
  spline S26 degree 2 poles (112.6216, 89.2589) (113.0805, 89.2589) (113.7721, 89.0812) (114.0694, 88.9519) knots 0 0 0 1 2 2 2
  line L80 (114.0694, 88.9519) -> (114.0694, 88.0018)
  line L81 (114.0694, 88.0018) -> (113.9789, 88.0018)
  spline S27 degree 2 poles (113.9789, 88.0018) (113.6784, 88.2571) (112.9577, 88.5318) (112.6184, 88.5318) knots 0 0 0 1 2 2 2
  spline S28 degree 2 poles (112.6184, 88.5318) (112.5311, 88.5318) (112.25, 88.493) (112.166, 88.4542) knots 0 0 0 1 2 2 2
  spline S29 degree 2 poles (112.166, 88.4542) (112.0626, 88.409) (111.9171, 88.2442) (111.9171, 88.1117) knots 0 0 0 1 2 2 2
  spline S30 degree 2 poles (111.9171, 88.1117) (111.9171, 87.9598) (112.153, 87.7724) (112.3146, 87.7304) knots 0 0 0 1 2 2 2
  spline S31 degree 2 poles (112.3146, 87.7304) (112.5182, 87.6754) (112.9803, 87.5817) (113.1839, 87.5106) knots 0 0 0 1 2 2 2
  spline S32 degree 2 poles (113.1839, 87.5106) (113.646, 87.349) (114.0468, 86.7964) (114.0468, 86.3828) knots 0 0 0 1 2 2 2
  spline S33 degree 2 poles (114.0468, 86.3828) (114.0468, 85.8237) (113.0999, 85.1289) (112.389, 85.1289) knots 0 0 0 1 2 2 2
  spline S34 degree 2 poles (112.389, 85.1289) (112.0335, 85.1289) (111.329, 85.2743) (111.0511, 85.3971) knots 0 0 0 1 2 2 2
  line L82 (111.0511, 85.3971) -> (111.0511, 86.3085)
  line L83 (111.0511, 86.3085) -> (111.1383, 86.3085)
  spline S35 degree 2 poles (111.1383, 86.3085) (111.3613, 86.1178) (112.0012, 85.856) (112.3372, 85.856) knots 0 0 0 1 2 2 2
  spline S36 degree 2 poles (112.3372, 85.856) (112.4697, 85.856) (112.6766, 85.8948) (112.7929, 85.9465) knots 0 0 0 1 2 2 2
  spline S37 degree 2 poles (112.7929, 85.9465) (112.8866, 85.9885) (113.0223, 86.1566) (113.0223, 86.26) knots 0 0 0 1 2 2 2
  spline S38 degree 2 poles (113.0223, 86.26) (113.0223, 86.4151) (112.8058, 86.5928) (112.4956, 86.6639) knots 0 0 0 1 2 2 2
  spline S39 degree 2 poles (112.4956, 86.6639) (112.2952, 86.7092) (111.9236, 86.7964) (111.7103, 86.8708) knots 0 0 0 1 2 2 2
  spline S40 degree 2 poles (111.7103, 86.8708) (111.2967, 87.0226) (110.8927, 87.5268) (110.8927, 87.9404) knots 0 0 0 1 2 2 2
  spline S41 degree 2 poles (110.8927, 87.9404) (110.8927, 88.535) (111.8267, 89.2589) (112.6216, 89.2589) knots 0 0 0 1 2 2 2
  line L84 (106.3071, 89.1878) -> (107.3024, 89.1878)
  line L85 (107.3024, 89.1878) -> (107.3024, 86.5444)
  line L86 (107.3024, 86.5444) -> (108.0263, 88.2507)
  line L87 (108.0263, 88.2507) -> (108.7114, 88.2507)
  line L88 (108.7114, 88.2507) -> (109.4353, 86.5444)
  line L89 (109.4353, 86.5444) -> (109.4353, 89.1878)
  line L90 (109.4353, 89.1878) -> (110.3789, 89.1878)
  line L91 (110.3789, 89.1878) -> (110.3789, 85.2)
  line L92 (110.3789, 85.2) -> (109.2252, 85.2)
  line L93 (109.2252, 85.2) -> (108.3398, 87.1681)
  line L94 (108.3398, 87.1681) -> (107.4608, 85.2)
  line L95 (107.4608, 85.2) -> (106.3071, 85.2)
  line L96 (106.3071, 85.2) -> (106.3071, 89.1878)
  line L97 (105.9096, 89.1878) -> (104.562, 85.2)
  line L98 (104.562, 85.2) -> (103.4697, 85.2)
  line L99 (103.4697, 85.2) -> (102.1221, 89.1878)
  line L100 (102.1221, 89.1878) -> (103.153, 89.1878)
  line L101 (103.153, 89.1878) -> (103.4019, 88.3735)
  line L102 (103.4019, 88.3735) -> (104.6557, 88.3735)
  line L103 (104.6557, 88.3735) -> (104.9078, 89.1878)
  line L104 (104.9078, 89.1878) -> (105.9096, 89.1878)
  line L105 (103.6216, 87.6496) -> (104.0288, 86.3311)
  line L106 (104.0288, 86.3311) -> (104.4392, 87.6496)
  line L107 (104.4392, 87.6496) -> (103.6216, 87.6496)
  line L108 (99.3527, 89.1878) -> (99.3527, 85.9594)
  line L109 (99.3527, 85.9594) -> (100.5322, 85.9594)
  line L110 (100.5322, 85.9594) -> (100.5322, 85.2)
  line L111 (100.5322, 85.2) -> (97.1713, 85.2)
  line L112 (97.1713, 85.2) -> (97.1713, 85.9594)
  line L113 (97.1713, 85.9594) -> (98.3509, 85.9594)
  line L114 (98.3509, 85.9594) -> (98.3509, 89.1878)
  line L115 (98.3509, 89.1878) -> (99.3527, 89.1878)
  line L116 (93.0769, 89.1878) -> (94.2952, 89.1878)
  line L117 (94.2952, 89.1878) -> (95.4036, 87.7239)
  line L118 (95.4036, 87.7239) -> (95.7656, 87.7239)
  line L119 (95.7656, 87.7239) -> (95.7656, 89.1878)
  line L120 (95.7656, 89.1878) -> (96.7609, 89.1878)
  line L121 (96.7609, 89.1878) -> (96.7609, 85.2)
  line L122 (96.7609, 85.2) -> (95.158, 85.2)
  spline S42 degree 2 poles (95.158, 85.2) (94.8252, 85.2) (94.334, 85.284) (94.1239, 85.4133) knots 0 0 0 1 2 2 2
  spline S43 degree 2 poles (94.1239, 85.4133) (93.9106, 85.549) (93.6586, 85.9724) (93.6586, 86.2955) knots 0 0 0 1 2 2 2
  spline S44 degree 2 poles (93.6586, 86.2955) (93.6586, 86.7512) (94.0722, 87.3232) (94.418, 87.4912) knots 0 0 0 1 2 2 2
  line L123 (94.418, 87.4912) -> (93.0769, 89.1878)
  spline S45 degree 2 poles (94.6862, 86.4216) (94.6862, 86.2697) (94.8026, 86.0532) (94.9351, 85.995) knots 0 0 0 1 2 2 2
  spline S46 degree 2 poles (94.9351, 85.995) (95.0288, 85.9562) (95.2582, 85.9336) (95.4295, 85.9336) knots 0 0 0 1 2 2 2
  line L124 (95.4295, 85.9336) -> (95.7656, 85.9336)
  line L125 (95.7656, 85.9336) -> (95.7656, 87.0065)
  line L126 (95.7656, 87.0065) -> (95.478, 87.0065)
  spline S47 degree 2 poles (95.478, 87.0065) (95.2711, 87.0065) (94.9771, 86.9548) (94.8769, 86.874) knots 0 0 0 1 2 2 2
  spline S48 degree 2 poles (94.8769, 86.874) (94.7799, 86.7964) (94.6862, 86.5896) (94.6862, 86.4216) knots 0 0 0 1 2 2 2
  line L127 (93.2094, 89.1878) -> (91.8618, 85.2)
  line L128 (91.8618, 85.2) -> (90.7695, 85.2)
  line L129 (90.7695, 85.2) -> (89.4219, 89.1878)
  line L130 (89.4219, 89.1878) -> (90.4528, 89.1878)
  line L131 (90.4528, 89.1878) -> (90.7017, 88.3735)
  line L132 (90.7017, 88.3735) -> (91.9555, 88.3735)
  line L133 (91.9555, 88.3735) -> (92.2076, 89.1878)
  line L134 (92.2076, 89.1878) -> (93.2094, 89.1878)
  line L135 (90.9214, 87.6496) -> (91.3286, 86.3311)
  line L136 (91.3286, 86.3311) -> (91.739, 87.6496)
  line L137 (91.739, 87.6496) -> (90.9214, 87.6496)
  line L138 (85.6086, 89.1878) -> (86.5717, 89.1878)
  line L139 (86.5717, 89.1878) -> (88.1099, 86.4086)
  line L140 (88.1099, 86.4086) -> (88.1099, 89.1878)
  line L141 (88.1099, 89.1878) -> (89.0245, 89.1878)
  line L142 (89.0245, 89.1878) -> (89.0245, 85.2)
  line L143 (89.0245, 85.2) -> (87.7964, 85.2)
  line L144 (87.7964, 85.2) -> (86.5232, 87.4848)
  line L145 (86.5232, 87.4848) -> (86.5232, 85.2)
  line L146 (86.5232, 85.2) -> (85.6086, 85.2)
  line L147 (85.6086, 85.2) -> (85.6086, 89.1878)
  spline S49 degree 2 poles (83.5663, 89.2589) (84.0252, 89.2589) (84.7167, 89.0812) (85.014, 88.9519) knots 0 0 0 1 2 2 2
  line L148 (85.014, 88.9519) -> (85.014, 88.0018)
  line L149 (85.014, 88.0018) -> (84.9235, 88.0018)
  spline S50 degree 2 poles (84.9235, 88.0018) (84.623, 88.2571) (83.9024, 88.5318) (83.563, 88.5318) knots 0 0 0 1 2 2 2
  spline S51 degree 2 poles (83.563, 88.5318) (83.4758, 88.5318) (83.1946, 88.493) (83.1106, 88.4542) knots 0 0 0 1 2 2 2
  spline S52 degree 2 poles (83.1106, 88.4542) (83.0072, 88.409) (82.8618, 88.2442) (82.8618, 88.1117) knots 0 0 0 1 2 2 2
  spline S53 degree 2 poles (82.8618, 88.1117) (82.8618, 87.9598) (83.0977, 87.7724) (83.2593, 87.7304) knots 0 0 0 1 2 2 2
  spline S54 degree 2 poles (83.2593, 87.7304) (83.4629, 87.6754) (83.925, 87.5817) (84.1286, 87.5106) knots 0 0 0 1 2 2 2
  spline S55 degree 2 poles (84.1286, 87.5106) (84.5907, 87.349) (84.9914, 86.7964) (84.9914, 86.3828) knots 0 0 0 1 2 2 2
  spline S56 degree 2 poles (84.9914, 86.3828) (84.9914, 85.8237) (84.0446, 85.1289) (83.3336, 85.1289) knots 0 0 0 1 2 2 2
  spline S57 degree 2 poles (83.3336, 85.1289) (82.9781, 85.1289) (82.2736, 85.2743) (81.9957, 85.3971) knots 0 0 0 1 2 2 2
  line L150 (81.9957, 85.3971) -> (81.9957, 86.3085)
  line L151 (81.9957, 86.3085) -> (82.083, 86.3085)
  spline S58 degree 2 poles (82.083, 86.3085) (82.3059, 86.1178) (82.9458, 85.856) (83.2819, 85.856) knots 0 0 0 1 2 2 2
  spline S59 degree 2 poles (83.2819, 85.856) (83.4144, 85.856) (83.6212, 85.8948) (83.7376, 85.9465) knots 0 0 0 1 2 2 2
  spline S60 degree 2 poles (83.7376, 85.9465) (83.8313, 85.9885) (83.967, 86.1566) (83.967, 86.26) knots 0 0 0 1 2 2 2
  spline S61 degree 2 poles (83.967, 86.26) (83.967, 86.4151) (83.7505, 86.5928) (83.4402, 86.6639) knots 0 0 0 1 2 2 2
  spline S62 degree 2 poles (83.4402, 86.6639) (83.2399, 86.7092) (82.8682, 86.7964) (82.655, 86.8708) knots 0 0 0 1 2 2 2
  spline S63 degree 2 poles (82.655, 86.8708) (82.2413, 87.0226) (81.8374, 87.5268) (81.8374, 87.9404) knots 0 0 0 1 2 2 2
  spline S64 degree 2 poles (81.8374, 87.9404) (81.8374, 88.535) (82.7713, 89.2589) (83.5663, 89.2589) knots 0 0 0 1 2 2 2
  line L152 (78.6542, 85.9594) -> (80.3282, 85.9594)
  line L153 (80.3282, 85.9594) -> (80.3282, 86.7124)
  line L154 (80.3282, 86.7124) -> (78.7867, 86.7124)
  line L155 (78.7867, 86.7124) -> (78.7867, 87.4718)
  line L156 (78.7867, 87.4718) -> (80.3282, 87.4718)
  line L157 (80.3282, 87.4718) -> (80.3282, 89.1878)
  line L158 (80.3282, 89.1878) -> (81.3235, 89.1878)
  line L159 (81.3235, 89.1878) -> (81.3235, 85.2)
  line L160 (81.3235, 85.2) -> (78.6542, 85.2)
  line L161 (78.6542, 85.2) -> (78.6542, 85.9594)
  spline S65 degree 2 poles (74.5081, 87.1939) (74.5081, 88.1634) (75.5422, 89.2718) (76.4406, 89.2718) knots 0 0 0 1 2 2 2
  spline S66 degree 2 poles (76.4406, 89.2718) (77.3422, 89.2718) (78.3699, 88.1505) (78.3699, 87.1939) knots 0 0 0 1 2 2 2
  spline S67 degree 2 poles (78.3699, 87.1939) (78.3699, 86.2341) (77.3422, 85.116) (76.4406, 85.116) knots 0 0 0 1 2 2 2
  spline S68 degree 2 poles (76.4406, 85.116) (75.5422, 85.116) (74.5081, 86.2277) (74.5081, 87.1939) knots 0 0 0 1 2 2 2
  spline S69 degree 2 poles (75.5422, 87.1939) (75.5422, 86.8352) (75.6876, 86.3343) (75.8137, 86.176) knots 0 0 0 1 2 2 2
  spline S70 degree 2 poles (75.8137, 86.176) (75.9397, 86.0112) (76.2628, 85.869) (76.4374, 85.869) knots 0 0 0 1 2 2 2
  spline S71 degree 2 poles (76.4374, 85.869) (76.6216, 85.869) (76.9221, 86.0015) (77.0611, 86.1695) knots 0 0 0 1 2 2 2
  spline S72 degree 2 poles (77.0611, 86.1695) (77.1839, 86.3246) (77.3357, 86.8384) (77.3357, 87.1939) knots 0 0 0 1 2 2 2
  spline S73 degree 2 poles (77.3357, 87.1939) (77.3357, 87.5623) (77.1903, 88.0471) (77.0643, 88.2119) knots 0 0 0 1 2 2 2
  spline S74 degree 2 poles (77.0643, 88.2119) (76.9383, 88.3767) (76.6119, 88.5189) (76.4374, 88.5189) knots 0 0 0 1 2 2 2
  spline S75 degree 2 poles (76.4374, 88.5189) (76.2596, 88.5189) (75.93, 88.367) (75.8104, 88.2054) knots 0 0 0 1 2 2 2
  spline S76 degree 2 poles (75.8104, 88.2054) (75.6812, 88.0309) (75.5422, 87.5688) (75.5422, 87.1939) knots 0 0 0 1 2 2 2
  line L162 (70.2294, 89.1878) -> (71.4478, 89.1878)
  line L163 (71.4478, 89.1878) -> (72.5562, 87.7239)
  line L164 (72.5562, 87.7239) -> (72.9181, 87.7239)
  line L165 (72.9181, 87.7239) -> (72.9181, 89.1878)
  line L166 (72.9181, 89.1878) -> (73.9135, 89.1878)
  line L167 (73.9135, 89.1878) -> (73.9135, 85.2)
  line L168 (73.9135, 85.2) -> (72.3106, 85.2)
  spline S77 degree 2 poles (72.3106, 85.2) (71.9777, 85.2) (71.4865, 85.284) (71.2765, 85.4133) knots 0 0 0 1 2 2 2
  spline S78 degree 2 poles (71.2765, 85.4133) (71.0632, 85.549) (70.8111, 85.9724) (70.8111, 86.2955) knots 0 0 0 1 2 2 2
  spline S79 degree 2 poles (70.8111, 86.2955) (70.8111, 86.7512) (71.2248, 87.3232) (71.5706, 87.4912) knots 0 0 0 1 2 2 2
  line L169 (71.5706, 87.4912) -> (70.2294, 89.1878)
  spline S80 degree 2 poles (71.8388, 86.4216) (71.8388, 86.2697) (71.9551, 86.0532) (72.0876, 85.995) knots 0 0 0 1 2 2 2
  spline S81 degree 2 poles (72.0876, 85.995) (72.1813, 85.9562) (72.4108, 85.9336) (72.5821, 85.9336) knots 0 0 0 1 2 2 2
  line L170 (72.5821, 85.9336) -> (72.9181, 85.9336)
  line L171 (72.9181, 85.9336) -> (72.9181, 87.0065)
  line L172 (72.9181, 87.0065) -> (72.6305, 87.0065)
  spline S82 degree 2 poles (72.6305, 87.0065) (72.4237, 87.0065) (72.1296, 86.9548) (72.0294, 86.874) knots 0 0 0 1 2 2 2
  spline S83 degree 2 poles (72.0294, 86.874) (71.9325, 86.7964) (71.8388, 86.5896) (71.8388, 86.4216) knots 0 0 0 1 2 2 2
  line L173 (65.8603, 89.1878) -> (66.8556, 89.1878)
  line L174 (66.8556, 89.1878) -> (66.8556, 86.5444)
  line L175 (66.8556, 86.5444) -> (67.5795, 88.2507)
  line L176 (67.5795, 88.2507) -> (68.2646, 88.2507)
  line L177 (68.2646, 88.2507) -> (68.9885, 86.5444)
  line L178 (68.9885, 86.5444) -> (68.9885, 89.1878)
  line L179 (68.9885, 89.1878) -> (69.9321, 89.1878)
  line L180 (69.9321, 89.1878) -> (69.9321, 85.2)
  line L181 (69.9321, 85.2) -> (68.7785, 85.2)
  line L182 (68.7785, 85.2) -> (67.893, 87.1681)
  line L183 (67.893, 87.1681) -> (67.014, 85.2)
  line L184 (67.014, 85.2) -> (65.8603, 85.2)
  line L185 (65.8603, 85.2) -> (65.8603, 89.1878)
  line L186 (65.033, 89.1878) -> (65.033, 85.2)
  line L187 (65.033, 85.2) -> (62.3379, 85.2)
  line L188 (62.3379, 85.2) -> (62.3379, 85.9594)
  line L189 (62.3379, 85.9594) -> (64.0377, 85.9594)
  line L190 (64.0377, 85.9594) -> (64.0377, 86.6607)
  line L191 (64.0377, 86.6607) -> (62.4704, 86.6607)
  line L192 (62.4704, 86.6607) -> (62.4704, 87.4201)
  line L193 (62.4704, 87.4201) -> (64.0377, 87.4201)
  line L194 (64.0377, 87.4201) -> (64.0377, 88.4284)
  line L195 (64.0377, 88.4284) -> (62.3379, 88.4284)
  line L196 (62.3379, 88.4284) -> (62.3379, 89.1878)
  line L197 (62.3379, 89.1878) -> (65.033, 89.1878)
  line L198 (57.9752, 89.1878) -> (59.1935, 89.1878)
  line L199 (59.1935, 89.1878) -> (60.302, 87.7239)
  line L200 (60.302, 87.7239) -> (60.6639, 87.7239)
  line L201 (60.6639, 87.7239) -> (60.6639, 89.1878)
  line L202 (60.6639, 89.1878) -> (61.6592, 89.1878)
  line L203 (61.6592, 89.1878) -> (61.6592, 85.2)
  line L204 (61.6592, 85.2) -> (60.0564, 85.2)
  spline S84 degree 2 poles (60.0564, 85.2) (59.7235, 85.2) (59.2323, 85.284) (59.0222, 85.4133) knots 0 0 0 1 2 2 2
  spline S85 degree 2 poles (59.0222, 85.4133) (58.809, 85.549) (58.5569, 85.9724) (58.5569, 86.2955) knots 0 0 0 1 2 2 2
  spline S86 degree 2 poles (58.5569, 86.2955) (58.5569, 86.7512) (58.9705, 87.3232) (59.3163, 87.4912) knots 0 0 0 1 2 2 2
  line L205 (59.3163, 87.4912) -> (57.9752, 89.1878)
  spline S87 degree 2 poles (59.5845, 86.4216) (59.5845, 86.2697) (59.7009, 86.0532) (59.8334, 85.995) knots 0 0 0 1 2 2 2
  spline S88 degree 2 poles (59.8334, 85.995) (59.9271, 85.9562) (60.1565, 85.9336) (60.3278, 85.9336) knots 0 0 0 1 2 2 2
  line L206 (60.3278, 85.9336) -> (60.6639, 85.9336)
  line L207 (60.6639, 85.9336) -> (60.6639, 87.0065)
  line L208 (60.6639, 87.0065) -> (60.3763, 87.0065)
  spline S89 degree 2 poles (60.3763, 87.0065) (60.1695, 87.0065) (59.8754, 86.9548) (59.7752, 86.874) knots 0 0 0 1 2 2 2
  spline S90 degree 2 poles (59.7752, 86.874) (59.6783, 86.7964) (59.5845, 86.5896) (59.5845, 86.4216) knots 0 0 0 1 2 2 2
  spline S91 degree 2 poles (52.5138, 87.1972) (52.5138, 87.7562) (53.0018, 88.6352) (53.3734, 88.8711) knots 0 0 0 1 2 2 2
  spline S92 degree 2 poles (53.3734, 88.8711) (53.6836, 89.0715) (54.414, 89.1878) (54.8244, 89.1878) knots 0 0 0 1 2 2 2
  line L209 (54.8244, 89.1878) -> (56.0718, 89.1878)
  line L210 (56.0718, 89.1878) -> (56.0718, 85.2)
  line L211 (56.0718, 85.2) -> (54.8373, 85.2)
  spline S93 degree 2 poles (54.8373, 85.2) (54.4172, 85.2) (53.6836, 85.3067) (53.3605, 85.5135) knots 0 0 0 1 2 2 2
  spline S94 degree 2 poles (53.3605, 85.5135) (52.9694, 85.7656) (52.5138, 86.6187) (52.5138, 87.1972) knots 0 0 0 1 2 2 2
  spline S95 degree 2 poles (53.5414, 87.1907) (53.5414, 86.7964) (53.8129, 86.2341) (54.0908, 86.0758) knots 0 0 0 1 2 2 2
  spline S96 degree 2 poles (54.0908, 86.0758) (54.2944, 85.9659) (54.7404, 85.9433) (55.0506, 85.9433) knots 0 0 0 1 2 2 2
  line L212 (55.0506, 85.9433) -> (55.07, 85.9433)
  line L213 (55.07, 85.9433) -> (55.07, 88.4413)
  line L214 (55.07, 88.4413) -> (55.0506, 88.4413)
  spline S97 degree 2 poles (55.0506, 88.4413) (54.7145, 88.4413) (54.2524, 88.4187) (54.0423, 88.2862) knots 0 0 0 1 2 2 2
  spline S98 degree 2 poles (54.0423, 88.2862) (53.7967, 88.1311) (53.5414, 87.5849) (53.5414, 87.1907) knots 0 0 0 1 2 2 2
  spline S99 degree 2 poles (50.2, 89.2654) (51.0983, 89.2654) (52.1518, 88.1796) (52.1518, 87.1972) knots 0 0 0 1 2 2 2
  spline S100 degree 2 poles (52.1518, 87.1972) (52.1518, 86.2503) (51.0951, 85.1225) (50.1967, 85.1225) knots 0 0 0 1 2 2 2
  spline S101 degree 2 poles (50.1967, 85.1225) (49.9608, 85.1225) (49.5795, 85.1774) (49.405, 85.2226) knots 0 0 0 1 2 2 2